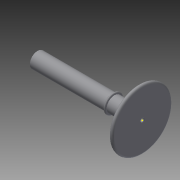
# Autodesk Inventor part: axilhollow
Saved by Autodesk Inventor 2015 (Build 190159000, 159)
## iProperties
Created: 2015-12-08
Part Number: axilhollow
Material: Generic
Document SubType Name: Modeling
Designer: Ross
Density: 1 g/cm^3
Appearance: Default
Author: Ross
Autodesk Inventor part; units mm, degrees
ref_plane "XY Plane" through (0, 0, 0) normal (0, 0, 1) x (1, 0, 0)
sketch "Sketch1" plane through (0, 0, 0) normal (0, 1, 0) x (-1, 0, 0)
  line L0 (0, 0) -> (50, 0)
  line L1 (0, 0) -> (0, 16)
  line L2 (0, 16) -> (2, 16)
  line L3 (2, 16) -> (2, 0)
  line L4 (2, 0) -> (2, 4.1)
  line L5 (50, 0) -> (50, 4.1)
  line L6 (50, 4.1) -> (2, 4.1)
  dimension "d0" = 50
  dimension "d1" = 16
  dimension "d2" = 2
  dimension "d3" = 4.1
  dimension "d4" = 4.1
  constraints: 14 end point, 2 perpendicular, 2 point on line, 2 vertical, 1 horizontal
  measures "d0" distance of L0.start L0.end
  measures "d1" distance of L0.start L1.end
  measures "d2" distance of L1.end L2.end
  measures "d3" distance of L3.end L4.end
  measures "d4" distance of L0.end L5.end
revolve "Revolution1" add sketch "Sketch1" angle 360 about axis through (0, 0, 0) along (-1, 0, 0)
sketch "Sketch2" plane through (0, 0, 0) normal (1, 0, 0) x (0, 0, -1)
  circle A0 centre (0, 0) radius 0.875
  dimension "d6" = 1.75
  constraints: 1 centre point, 1 coincident
  measures "d6" diameter of A0
extrude "Extrusion1" cut sketch "Sketch2" against normal blind 8
fillet "Fillet1" radius 0.3 1 edges at (0, 0, 0.875)
ref_plane "Work Plane1" through (-15, 0, 0) normal (1, 0, 0) x (0, 1, 0)
sketch "Sketch3" plane through (-15, 0, 0) normal (1, 0, 0) x (0, 1, 0)
  line L0 (0, 0) -> (-5.6972, 0)
  circle A0 centre (0, 0) radius 5
  dimension "d11" = 10
  constraints: 2 end point, 1 centre point, 1 coincident, 1 horizontal
  measures "d11" diameter of A0
extrude "Extrusion2" add sketch "Sketch3" against normal blind 1
fillet "Fillet2" radius 0.5 2 edges at (-16, -5, 0) (-15, -5, 0)
ref_plane "Work Plane2" through (-16, 0, 0) normal (1, 0, 0) x (0, 1, 0)
sketch "Sketch4" plane through (-50, 0, 0) normal (-1, 0, 0) x (0, 0, 1)
  circle A0 centre (0, 0) radius 4.1
  constraints: 1 centre point, 1 coincident
extrude "Extrusion3" add sketch "Sketch4" along normal blind 10
ref_plane "Work Plane3" through (0, 0, 0) normal (0, 1, 0) x (-1, 0, 0)
sketch "Sketch5" plane through (0, 0, 0) normal (0, 1, 0) x (-1, 0, 0)
  point P0 (0, 0)
sketch "Sketch6" plane through (-60, 0, 0) normal (-1, 0, 0) x (0, 0, 1)
  circle A0 centre (0, 0) radius 4.1
  constraints: 1 centre point, 1 coincident
extrude "Extrusion4" cut sketch "Sketch6" against normal blind 8
sketch "Sketch7" plane through (-52, 0, 0) normal (-1, 0, 0) x (0, 0, 1)
  circle A0 centre (0, 0) radius 4.1
  constraints: 1 centre point, 1 coincident
extrude "Extrusion5" add sketch "Sketch7" along normal blind 4
sketch "Sketch8" plane through (0, 0, 0) normal (0, 1, 0) x (-1, 0, 0)
  point P0 (0, 0)
sketch "Sketch9" plane through (-56, 0, 0) normal (-1, 0, 0) x (0, 0, 1)
  circle A0 centre (0, 0) radius 0.875 projected
  circle A1 centre (0, 0) radius 3.7
  dimension "d28" = 7.4
  constraints: 1 centre point, 1 coincident
  measures "d28" diameter of A1
extrude "Extrusion7" cut sketch "Sketch9" against normal blind 47 contours A0 | A1
sketch "Sketch10" plane through (-9, 0, 0) normal (-1, 0, 0) x (0, 0, 1)
  circle A0 centre (0, 0) radius 3.7
  circle A1 centre (0, 0) radius 1.25
  dimension "d31" = 2.5
  constraints: 2 centre point, 2 coincident
  measures "d31" diameter of A1
extrude "Extrusion8" cut sketch "Sketch10" against normal blind 8
fillet "Fillet3" radius 0.5 1 edges at (-9, 0, -1.25)
fillet "Fillet4" radius 1 2 edges at (-2, 0, -16) (0, 0, -16)
body "Solid1"
